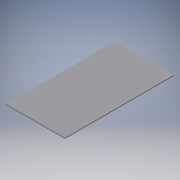
# Autodesk Inventor part: EinschubRechts
Saved by Autodesk Inventor 2018 (Build 220112000, 112)
## iProperties
Created: 2017-11-12
Part Number: EinschubRechts
Material: Generisch
Document SubType Name: Blech
Density: 1 g/cm^3
Sheet Metal Rule: Standard_mm
Appearance: Vorgabe
Autodesk Inventor part; units mm, degrees
ref_plane "YZ Plane" through (0, 0, 0) normal (1, 0, 0) x (0, 1, 0)
ref_plane "XZ Plane" through (0, 0, 0) normal (0, 1, 0) x (-1, 0, 0)
ref_plane "XY Plane" through (0, 0, 0) normal (0, 0, 1) x (1, 0, 0)
sketch "Skizze1" plane through (0, 0, 0) normal (0, 0, 1) x (1, 0, 0)
  line L0 (-273, 285) -> (68, 285)
  line L1 (68, -8) -> (-273, -8)
  line L2 (5, 153.9294) -> (5, 157.0706)
  line L3 (5, 253.9294) -> (5, 257.0706)
  line L4 (0, 285) -> (-235, 285)
  line L5 (-235, 285) -> (-235, -8)
  line L6 (-235, -8) -> (0, -8)
  line L7 (0, -8) -> (0, 285)
  line L8 (-199.0415, -3.8) -> (-199.0415, -6)
  line L9 (-138, 2) -> (-138, 4.5)
  line L10 (-250, 282.9) -> (-250, -5.9)
  point P0 (0, 0)
  point P1 (-273, -8)
  dimension "d0" = 5
  dimension "d1" = 0
  dimension "d2" = 0
  dimension "d15" = 15
  measures "d0" distance between parallel lines of L3 L7
  measures "d1" distance between parallel lines of L0 L4
  measures "d2" vertical extent of L6
  measures "d15" distance between parallel lines of L10 L5
extrude "Grobblech1" add sketch "Skizze1" along normal blind 2
sketch "Skizze2" plane through (-235, -6, 2) normal (0, -1, 0) x (1, 0, 0)
  line L0 (235, 0) -> (0, 0)
  line L1 (0, 0) -> (0, -18)
  line L2 (0, -18) -> (235, -18)
  line L3 (235, -18) -> (235, 0)
  constraints: 6 end point, 1 horizontal, 1 perpendicular, 1 vertical
edge flange "Lasche1" height 18 angle 90 thickness 2 bend radius 2 thickness toward (0, -1, 0) relief tear relief width 2 relief depth 1 corner gap 2 corner form 0 edges at (-117.5, -8, 0) (-117.5, 285, 0) wall of the first edge with corners at (0, -6, 2) (-235, -6, 2) (-235, -6, -16) (0, -6, -16)
bend "Biegung1"
corner "Ecke1"
sketch "Skizze3" plane through (0, 0, 2) normal (0, 0, 1) x (1, 0, 0)
  line L0 (-273, 285) -> (68, 285) construction
  line L1 (0, 281) -> (0, -4) construction
  line L2 (0, 281) -> (0, 285) construction
  line L3 (0, -8) -> (0, -4) construction
  line L4 (68, -8) -> (-273, -8) construction
  line L5 (-235, -4) -> (-235, 281) construction
  line L6 (-235, 285) -> (-235, 281) construction
  line L7 (-235, -4) -> (-235, -8) construction
  line L8 (-250, 282.9) -> (-250, -5.9) construction
  line L9 (-225, 285) -> (-225, -8) construction
  line L10 (0, -8) -> (-235, -8) projected
  line L11 (-225, 285) -> (-217, 285)
  line L12 (-217, 285) -> (-217, -8)
  line L13 (-217, -8) -> (-225, -8)
  line L14 (-225, -8) -> (-225, 285)
  point P0 (0, 0)
  dimension "d16" = 25
  dimension "d17" = 8
  dimension "d18" = 293
  constraints: 10 end point, 3 point on line, 2 parallel, 2 perpendicular, 1 horizontal, 1 vertical
  measures "d16" distance between parallel lines of L8 L9
  measures "d17" distance of L12.end L13.end
  measures "d18" distance of L11.end L12.end
extrude "Extrusion1" cut sketch "Skizze3" against normal blind 4.75
equation "\"d4\" = Stärke"
equation "\"d5\" = BreiteBiegungsfreistellung"
equation "\"d6\" = TiefeBiegungsfreistellung"
equation "\"d7\" = MinimalRest"
equation "\"d8\" = Übergangsradius"
equation "\"d11\" = Biegeradius"
equation "\"d12\" = GrößeEckenfreistellung"
equation "\"d13\" = Abstandsgröße"
equation "\"d14\" = JacobiRadiusGröße"
equation "\"Biegeradius\" = Stärke"
equation "\"BreiteBiegungsfreistellung\" = Stärke"
equation "\"TiefeBiegungsfreistellung\" = 0.5 * Stärke"
equation "\"GrößeEckenfreistellung\" = 4 * Stärke"
equation "\"MinimalRest\" = 2 * Stärke"
equation "\"Übergangsradius\" = Biegeradius"
equation "\"JacobiRadiusGröße\" = Biegeradius"
equation "\"Abstandsgröße\" = Stärke"
equation "\"Stärke\" = 2"
